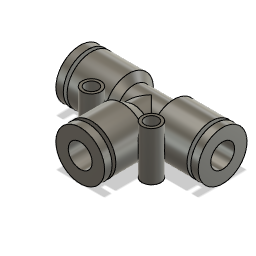
Bottom+Hydraulic+Assembly (Autodesk Fusion 360 archive; units mm, degrees)
design "Marine 3-Way Push-to-Connect"
Autodesk Fusion 360 part; units mm, degrees
sketch "Sketch1" plane through (0, 0, 0) normal (0, 1, 0) x (1, 0, 0)
  line L0 (0, -20) -> (0, -2.5)
  line L1 (0, 3.18) -> (19, 3.18)
  line L2 (2.5, 0) -> (20, 0)
  line L3 (19, 3.18) -> (19, 6.5)
  line L4 (0, 4.55) -> (4.65, 4.55)
  line L5 (4.65, 4.55) -> (6, 6.5)
  line L6 (17, 6.5) -> (17, 3.75)
  line L7 (17, 3.75) -> (16, 3.75)
  line L8 (16, 3.75) -> (16, 6.5)
  line L9 (19, 6.5) -> (17, 6.5)
  line L10 (16, 6.5) -> (6, 6.5)
  line L11 (0, 4.55) -> (-4.65, 4.55)
  line L12 (0, 3.18) -> (-19, 3.18)
  line L13 (-4.65, 4.55) -> (-6, 6.5)
  line L14 (-16, 6.5) -> (-6, 6.5)
  line L15 (-16, 3.75) -> (-16, 6.5)
  line L16 (-17, 6.5) -> (-17, 3.75)
  line L17 (-17, 3.75) -> (-16, 3.75)
  line L18 (-19, 6.5) -> (-17, 6.5)
  line L19 (-19, 3.18) -> (-19, 6.5)
  dimension "d2" = 19
  dimension "d3" = 3.18
  dimension "d4" = 6.5
  dimension "d5" = 6
  dimension "d6" = 4.65
  dimension "d7" = 4.55
  dimension "d8" = 1
  dimension "d9" = 2
  dimension "d10" = 2.75
  constraint horizontal L1
  constraint coincident L0 L1.start
  constraint perpendicular L1 L3
  constraint perpendicular L3 L9
  constraint horizontal L4
  constraint perpendicular L6 L9
  constraint perpendicular L3 L7
  constraint coincident L8.end L9
  constraint perpendicular L8 L9
  constraint collinear L9 L10
  constraint symmetric L0 L1.start L12.start
  constraint symmetric L0 L1.end L12.end
  constraint symmetric L0 L3.end L18.start
  constraint symmetric L0 L5.end L13.end
  constraint symmetric L0 L4.start L11.start
  constraint symmetric L0 L4.end L11.end
  constraint symmetric L0 L6.start L16.start
  constraint symmetric L0 L6.end L16.end
  constraint symmetric L0 L7.end L15.start
  constraint symmetric L0 L8.end L14.start
  constraint coincident L4.start L11.start
  measures "d2" distance of L1.start L1.end
  measures "d3" distance of L1 L2
  measures "d4" distance of L2 L3.end
  measures "d5" distance of L0 L5.end
  measures "d6" distance of L4.start L4.end
  measures "d7" distance of L2 L4
  measures "d8" distance of L6.end L7.end
  measures "d9" distance of L3.end L6.start
  measures "d10" distance of L6.start L6.end
revolve "Revolve1" add sketch "Sketch1" angle 360 about axis through (2.5, 0, 0) along (1, 0, 0)
sketch "Sketch2" plane through (0, 0, 0) normal (0, 1, 0) x (1, 0, 0)
  line L0 (3.75, -16) -> (6.5, -16)
  line L1 (3.18, -19) -> (6.5, -19)
  line L2 (4.55, -4.65) -> (6.5, -7.75)
  line L3 (4.55, 0) -> (4.55, -4.65)
  line L4 (3.18, 0) -> (3.18, -19)
  line L5 (6.5, -17) -> (3.75, -17)
  line L6 (6.5, -19) -> (6.5, -17)
  line L7 (6.5, -16) -> (6.5, -7.75)
  line L8 (3.75, -17) -> (3.75, -16)
  line L9 (0, -20) -> (0, -2.5)
  line L10 (4.55, 0) -> (3.18, 0)
  line L11 (2.5, 0) -> (20, 0)
  dimension "d12" = 19
  dimension "d13" = 4.65
  dimension "d14" = 1
  dimension "d15" = 2
  dimension "d16" = 2.75
  dimension "d17" = 3.18
  dimension "d18" = 6.5
  dimension "d19" = 4.55
  dimension "d20" = 8.25
  constraint perpendicular L1 L4
  constraint perpendicular L1 L6
  constraint perpendicular L5 L6
  constraint perpendicular L1 L8
  constraint coincident L0.end L6
  constraint perpendicular L0 L6
  constraint collinear L6 L7
  constraint parallel L4 L9
  constraint perpendicular L3 L10
  constraint coincident L4.start L11
  measures "d12" distance of L1.start L4.start
  measures "d13" distance of L3.start L2.start
  measures "d14" distance of L0.start L5.end
  measures "d15" distance of L5.start L1.end
  measures "d16" distance of L5.start L5.end
  measures "d17" distance of L4 L9
  measures "d18" distance of L7 L9
  measures "d19" distance of L3 L9
  measures "d20" distance of L2.end L0.end
revolve "Revolve2" add sketch "Sketch2" angle 360 about axis through (0, 0, 20) along (0, 0, -1)
sketch "Sketch3" plane through (19, 0, 0) normal (1, 0, 0) x (0, 0, -1)
  circle A0 centre (0, 0) radius 6.5
  circle A1 centre (0, 0) radius 3.18
  circle A2 centre (0, 0) radius 3.18
extrude "Extrude1" cut sketch "Sketch3" against normal up to surface (38 mm away) contours A1 A2
sketch "Sketch4" plane through (0, 0, 19) normal (0, 0, 1) x (1, 0, 0)
  circle A0 centre (0, 0) radius 6.5
  circle A1 centre (0, 0) radius 3.18
  circle A2 centre (0, 0) radius 3.18
extrude "Extrude2" cut sketch "Sketch4" along normal up to surface contours A1 A2 end surface at (-12.6667, 3.1455, -0.4668)
ref_plane "WorkPlane1" through (0, 6.5, 0) normal (0, 1, 0) x (0, 0, 1)
sketch "Sketch5" plane through (0, 6.5, 0) normal (0, 1, 0) x (1, 0, 0)
  line L0 (0, -20) -> (0, -2.5)
  line L1 (2.5, 0) -> (20, 0)
  circle A0 centre (8, -8) radius 1.75
  circle A1 centre (8, -8) radius 2.5
  circle A2 centre (-8, -8) radius 2.5
  circle A3 centre (-8, -8) radius 1.75
  dimension "d27" = 8
  dimension "d28" = 8
  dimension "d29" = 3.5
  dimension "d30" = 5
  constraint concentric A0 A1
  constraint symmetric L0 A0 A3
  constraint symmetric L0 A1 A2
  measures "d27" distance of L1 A0.centre
  measures "d28" distance of L0 A0.centre
  measures "d29" diameter of A0
  measures "d30" diameter of A1
extrude "Extrude3" add sketch "Sketch5" against normal blind 13
extrude "Extrude4" cut sketch "Sketch5" against normal up to surface (13 mm away) contours A0 | A3
